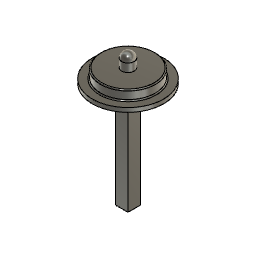
thomas_train_car_wheel v8 (Autodesk Fusion 360 design; units mm, degrees)
Autodesk Fusion 360 part; units mm, degrees
sketch "Sketch1" plane through (0, 0, 0) normal (0, 0, 1) x (1, 0, 0) in component "wheel"
  circle A0 centre (0, 0) radius 8.6
  dimension "d9" = 17.2
  constraint coincident A0.centre origin
  measures "d9" diameter of A0
extrude "Extrude1" add sketch "Sketch1" along normal blind 1 makes body 1 in component "wheel"
sketch "Sketch2" plane through (0, 0, 1) normal (0, 0, 1) x (-1, 0, 0) in component "wheel"
  circle A0 centre (0, 0) radius 8.6
  circle A1 centre (0, 0) radius 6.6
  dimension "d13" = 13.2
  constraint concentric A0 A1
  measures "d13" diameter of A1
extrude "Extrude2" add sketch "Sketch2" along normal blind 2.3 contours A1 bodies 1 in component "wheel"
sketch "Sketch3" plane through (0, 0, 3.3) normal (0, 0, 1) x (-1, 0, 0) in component "wheel"
  circle A0 centre (0, 0) radius 6.6
  circle A1 centre (0, 0) radius 1.5
  dimension "d16" = 3
  constraint coincident A0.centre A1.centre
  measures "d16" diameter of A1
extrude "Extrude3" add sketch "Sketch3" along normal blind 3.5 contours A1 bodies 1 in component "wheel"
fillet "Fillet1" radius 1.5 1 edges at (1.3985, 0.5424, 6.8) on bodies 1 in component "wheel"
fillet "Fillet2" radius 0.25 2 edges at (6.1534, -2.3867, 1) (6.1534, 2.3867, 3.3) on bodies 1 in component "wheel"
sketch "Sketch4" plane through (0, 0, 0) normal (0, 0, -1) x (1, 0, 0) in component "wheel"
  circle A0 centre (0, 0) radius 8.6
  line L0 (0.5, -0.5) -> (-0.5, 0.5) construction
  line L1 (-2.0512, -2.0678) -> (2.0552, 2.0719) construction
  circle A1 centre (0, 0) radius 1.5
  dimension "d19" = 3
  dimension "d20" = 3
  dimension "d32" = 3
  constraint coincident L0 A0.centre
  constraint coincident L1 A0.centre
  constraint coincident A0.centre A1.centre
  measures "d19" distance of L0.end L1.end
  measures "d20" distance of L1.start L0.end
  measures "d32" diameter of A1
sketch "Sketch1 (2)" plane through (0, 0, 0) normal (0, 0, -1) x (1, 0, 0)
  circle A0 centre (0, 0) radius 8.6
  line L0 (1.625, -1.625) -> (-1.625, -1.625)
  line L1 (-1.625, -1.625) -> (-1.625, 1.625)
  line L2 (-1.625, 1.625) -> (1.625, 1.625)
  line L3 (1.625, 1.625) -> (1.625, -1.625)
  line L4 (1.625, -1.625) -> (-1.625, 1.625) construction
  line L5 (-1.625, -1.625) -> (1.625, 1.625) construction
  dimension "d33" = 3.25
  dimension "d34" = 3.25
  constraint horizontal L0
  constraint perpendicular L0 L1
  constraint parallel L0 L2
  constraint parallel L1 L3
  constraint coincident L4 A0.centre
  constraint coincident L5 A0.centre
  constraint coincident A0.centre origin
  measures "d33" distance of L1.end L2.end
  measures "d34" distance of L0.end L1.end
extrude "Extrude6" cut sketch "Sketch1 (2)" against normal blind 2 contours L0 L1 L2 L3 bodies 1 in component "wheel"
sketch "Sketch1 (3)" plane through (0, 0, 2) normal (0, 0, -1) x (1, 0, 0) in component "pin"
  line L0 (1.625, 1.625) -> (-1.625, 1.625)
  line L1 (-1.625, 1.625) -> (-1.625, -1.625)
  line L2 (-1.625, -1.625) -> (1.625, -1.625)
  line L3 (1.625, -1.625) -> (1.625, 1.625)
  line L4 (-1.5, -1.5) -> (1.5, -1.5)
  line L5 (1.5, -1.5) -> (1.5, 1.5)
  line L6 (1.5, 1.5) -> (-1.5, 1.5)
  line L7 (-1.5, 1.5) -> (-1.5, -1.5)
  line L8 (-1.5, -1.5) -> (1.5, 1.5) construction
  line L9 (1.5, -1.5) -> (-1.5, 1.5) construction
  dimension "d40" = 3
  dimension "d41" = 3
  constraint horizontal L4
  constraint perpendicular L4 L5
  constraint parallel L4 L6
  constraint parallel L5 L7
  constraint coincident L8 origin
  constraint coincident L9 origin
  measures "d40" distance of L5.end L6.end
  measures "d41" distance of L4.end L5.end
extrude "Extrude2'" add sketch "Sketch1 (3)" along normal blind 27.5 separate body contours L4 L5 L6 L7 makes body 2 in component "pin"
component "wheel" placed x (1, 0, 0) y (0, 1, 0) z (0, 0, 1) at (0, 0, 0)
component "pin" placed x (1, 0, 0) y (0, 1, 0) z (0, 0, 1) at (0, 0, 0)
equation "outer_wheel_diameter = 17.2 mm"
equation "outer_lip = 2 mm"
equation "inner_wheel_diameter = 13.2 mm"
equation "inner_wheel_height = 2.3 mm"
equation "peg_diameter = 3 mm"
equation "peg_height = 3.5 mm"
equation "pin_side = 3 mm"
equation "pin_depth = 2 mm"
equation "d9 = outer_wheel_diameter"
equation "outer_wheel_thickness = 1 mm"
equation "d11 = outer_wheel_thickness"
equation "d13 = inner_wheel_diameter"
equation "d14 = inner_wheel_height"
equation "d16 = peg_diameter"
equation "d17 = peg_height"
equation "d19 = pin_side"
equation "d20 = pin_side"
equation "distance_between_wheels = 23.5 mm"
equation "d26 = peg_diameter / 2"
equation "pin_diameter = 3 mm"
equation "d32 = pin_diameter"
equation "d33 = pin_side + wheel_pin_tolerance"
equation "d34 = pin_side + wheel_pin_tolerance"
equation "d35 = -pin_depth"
equation "wheel_pin_tolerance = 0.25 mm"
equation "d40 = pin_side"
equation "d41 = pin_side"
equation "d42 = pin_depth * 2 + distance_between_wheels"
